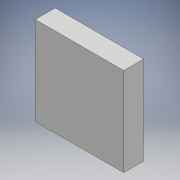
# Autodesk Inventor part: 球底座
Saved by Autodesk Inventor 2017 (Build 210142000, 142)
## iProperties
Created: 2021-05-18
Part Number: 球底座
Material: Generic
Document SubType Name: Modeling
Designer: user
Density: 1 g/cm^3
Appearance: Default
Author: user
Autodesk Inventor part; units mm, degrees
ref_plane "YZ Plane" through (0, 0, 0) normal (1, 0, 0) x (0, 1, 0)
ref_plane "XZ Plane" through (0, 0, 0) normal (0, 1, 0) x (-1, 0, 0)
sketch "Sketch1" plane through (0, 0, 0) normal (0, 1, 0) x (-1, 0, 0)
  line L0 (0, 0) -> (-400, 0)
  line L1 (-400, 0) -> (-400, -400)
  line L2 (-400, -400) -> (0, -400)
  line L3 (0, -400) -> (0, 0)
  dimension "d0" = 400
  dimension "d1" = 400
  constraints: 8 end point, 2 parallel, 1 horizontal, 1 perpendicular
  measures "d0" distance of L1.end L2.end
  measures "d1" distance of L2.end L0.start
extrude "Extrusion1" add sketch "Sketch1" along normal blind 20
ref_plane "Work Plane1" through (0, 0, -50) normal (0, 0, 1) x (1, 0, 0)
sketch "Sketch2" plane through (0, 0, -50) normal (0, 0, 1) x (1, 0, 0)
  line L0 (0, 20) -> (400, 20) projected
  arc A0 (4.9134, 69) -> (50, 25) centre (50, 70.1) ccw
  line L1 (50, 25) -> (50, 20)
  line L2 (0, 20) -> (50, 20)
  line L3 (50, 70.1) -> (50, 25)
  line L4 (0, 0) -> (0, 20) projected
  line L5 (0, 20) -> (0, 73.9134)
  line L6 (0, 73.9134) -> (4.9134, 69)
  dimension "d5" = 45.1
  dimension "d6" = 50
  dimension "d7" = 5
  dimension "d15" = 44
  dimension "d16" = 45
  constraints: 10 end point, 3 point on circle, 2 vertical, 1 centre point, 1 collinear, 1 perpendicular, 1 point on line
  measures "d5" radius of A0
  measures "d6" distance between parallel lines of L4 L1
  measures "d7" distance of L1.end L1.start
  measures "d15" vertical distance of L6.end L1.start
  measures "d16" angle of L5 L6
revolve "Revolution1" add sketch "Sketch2" angle 360 about axis through (50, 25, -50) along (0, -1, 0)
pattern_linear "Rectangular Pattern1" count 4 spacing 100 along (1, 0, 0) count 4 spacing -100 along (0, 0, 1) of "Revolution1"
sketch "Sketch4" plane through (0, 20, 0) normal (0, 1, 0) x (1, 0, 0)
  arc A0 (50, 100) -> (100, 150) centre (50, 150) ccw projected
  arc A1 (100, 50) -> (50, 100) centre (50, 50) ccw projected
  arc A2 (150, 100) -> (100, 50) centre (150, 50) ccw projected
  arc A3 (100, 150) -> (150, 100) centre (150, 150) ccw projected
  arc A4 (100, 250) -> (150, 200) centre (150, 250) ccw projected
  arc A5 (50, 200) -> (100, 250) centre (50, 250) ccw projected
  arc A6 (100, 150) -> (50, 200) centre (50, 150) ccw projected
  arc A7 (150, 200) -> (100, 150) centre (150, 150) ccw projected
  arc A8 (50, 200) -> (0, 150) centre (50, 150) ccw projected
  arc A9 (0, 250) -> (50, 200) centre (50, 250) ccw projected
  line L0 (0, 250) -> (0, 150) projected
  arc A10 (0, 150) -> (50, 100) centre (50, 150) ccw projected
  line L1 (0, 150) -> (0, 50) projected
  arc A11 (50, 100) -> (0, 50) centre (50, 50) ccw projected
  arc A12 (0, 50) -> (50, 0) centre (50, 50) ccw projected
  line L2 (0, 50) -> (0, 0) projected
  line L3 (0, 0) -> (50, 0) projected
  arc A13 (50, 300) -> (0, 250) centre (50, 250) ccw projected
  arc A14 (0, 350) -> (50, 300) centre (50, 350) ccw projected
  line L4 (0, 350) -> (0, 250) projected
  arc A15 (50, 400) -> (0, 350) centre (50, 350) ccw projected
  line L5 (50, 400) -> (0, 400) projected
  line L6 (0, 400) -> (0, 350) projected
  arc A16 (100, 350) -> (50, 400) centre (50, 350) ccw projected
  arc A17 (150, 400) -> (100, 350) centre (150, 350) ccw projected
  line L7 (150, 400) -> (50, 400) projected
  arc A18 (100, 350) -> (150, 300) centre (150, 350) ccw projected
  arc A19 (50, 300) -> (100, 350) centre (50, 350) ccw projected
  arc A20 (100, 250) -> (50, 300) centre (50, 250) ccw projected
  arc A21 (150, 300) -> (100, 250) centre (150, 250) ccw projected
  arc A22 (200, 350) -> (250, 300) centre (250, 350) ccw projected
  arc A23 (150, 300) -> (200, 350) centre (150, 350) ccw projected
  arc A24 (200, 250) -> (150, 300) centre (150, 250) ccw projected
  arc A25 (250, 300) -> (200, 250) centre (250, 250) ccw projected
  arc A26 (200, 250) -> (250, 200) centre (250, 250) ccw projected
  arc A27 (150, 200) -> (200, 250) centre (150, 250) ccw projected
  arc A28 (200, 150) -> (150, 200) centre (150, 150) ccw projected
  arc A29 (250, 200) -> (200, 150) centre (250, 150) ccw projected
  arc A30 (200, 150) -> (250, 100) centre (250, 150) ccw projected
  arc A31 (150, 100) -> (200, 150) centre (150, 150) ccw projected
  arc A32 (200, 50) -> (150, 100) centre (150, 50) ccw projected
  arc A33 (250, 100) -> (200, 50) centre (250, 50) ccw projected
  arc A34 (150, 0) -> (200, 50) centre (150, 50) ccw projected
  line L8 (150, 0) -> (250, 0) projected
  arc A35 (200, 50) -> (250, 0) centre (250, 50) ccw projected
  arc A36 (300, 150) -> (350, 100) centre (350, 150) ccw projected
  arc A37 (250, 100) -> (300, 150) centre (250, 150) ccw projected
  arc A38 (300, 50) -> (250, 100) centre (250, 50) ccw projected
  arc A39 (350, 100) -> (300, 50) centre (350, 50) ccw projected
  arc A40 (250, 0) -> (300, 50) centre (250, 50) ccw projected
  line L9 (250, 0) -> (350, 0) projected
  arc A41 (300, 50) -> (350, 0) centre (350, 50) ccw projected
  arc A42 (350, 0) -> (400, 50) centre (350, 50) ccw projected
  line L10 (350, 0) -> (400, 0) projected
  line L11 (400, 0) -> (400, 50) projected
  arc A43 (350, 100) -> (400, 150) centre (350, 150) ccw projected
  arc A44 (400, 50) -> (350, 100) centre (350, 50) ccw projected
  line L12 (400, 50) -> (400, 150) projected
  arc A45 (350, 200) -> (400, 250) centre (350, 250) ccw projected
  arc A46 (400, 150) -> (350, 200) centre (350, 150) ccw projected
  line L13 (400, 150) -> (400, 250) projected
  arc A47 (350, 200) -> (300, 150) centre (350, 150) ccw projected
  arc A48 (300, 250) -> (350, 200) centre (350, 250) ccw projected
  arc A49 (250, 200) -> (300, 250) centre (250, 250) ccw projected
  arc A50 (300, 150) -> (250, 200) centre (250, 150) ccw projected
  arc A51 (350, 300) -> (300, 250) centre (350, 250) ccw projected
  arc A52 (300, 350) -> (350, 300) centre (350, 350) ccw projected
  arc A53 (250, 300) -> (300, 350) centre (250, 350) ccw projected
  arc A54 (300, 250) -> (250, 300) centre (250, 250) ccw projected
  arc A55 (300, 350) -> (250, 400) centre (250, 350) ccw projected
  arc A56 (350, 400) -> (300, 350) centre (350, 350) ccw projected
  line L14 (350, 400) -> (250, 400) projected
  arc A57 (200, 350) -> (150, 400) centre (150, 350) ccw projected
  arc A58 (250, 400) -> (200, 350) centre (250, 350) ccw projected
  line L15 (250, 400) -> (150, 400) projected
  arc A59 (400, 350) -> (350, 400) centre (350, 350) ccw projected
  line L16 (400, 350) -> (400, 400) projected
  line L17 (400, 400) -> (350, 400) projected
  arc A60 (350, 300) -> (400, 350) centre (350, 350) ccw projected
  arc A61 (400, 250) -> (350, 300) centre (350, 250) ccw projected
  line L18 (400, 250) -> (400, 350) projected
  arc A62 (100, 50) -> (150, 0) centre (150, 50) ccw projected
  arc A63 (50, 0) -> (100, 50) centre (50, 50) ccw projected
  line L19 (50, 0) -> (150, 0) projected
extrude "Extrusion2" add sketch "Sketch4" along normal blind 48 contours A0 A3 A2 A1 | A11 L1 A10 | A6 A5 A4 A7 | A62 L19 A63 | L0 A9 A8 | A12 L3 L2 | A31 A30 A33 A32 | A27 A26 A29 A28 | A34 A35 L8 | L4 A14 A13 | A20 A19 A18 A21 | A24 A23 A22 A25 | A40 A41 L9 | L6 L5 A15 | A49 A48 A47 A50 | A37 A36 A39 A38 | A53 A52 A51 A54 | A42 L11 L10 | A16 L7 A17 | A57 L15 A58 | A55 L14 A56 | A43 L12 A44 | A45 L13 A46 | A60 L18 A61 | L17 L16 A59
sketch "Sketch5" plane through (0, 0, 0) normal (0, -1, 0) x (1, 0, 0)
  line L0 (-40, 40) -> (440, 40)
  line L1 (440, 40) -> (440, -440)
  line L2 (440, -440) -> (-40, -440)
  line L3 (-40, -440) -> (-40, 40)
  line L4 (400, 0) -> (400, -400) projected
  line L5 (400, -400) -> (0, -400) projected
  line L6 (0, 0) -> (400, 0) projected
  line L7 (0, -400) -> (0, 0) projected
  dimension "d20" = 40
  dimension "d21" = 40
  dimension "d22" = 40
  dimension "d23" = 40
  constraints: 8 end point, 2 parallel, 1 horizontal, 1 perpendicular
  measures "d20" distance between parallel lines of L1 L4
  measures "d21" distance between parallel lines of L2 L5
  measures "d22" distance between parallel lines of L0 L6
  measures "d23" distance between parallel lines of L3 L7
extrude "Extrusion3" add sketch "Sketch5" against normal up to surface (68 mm away)
sketch "Sketch6" plane through (0, 0, 0) normal (0, -1, 0) x (1, 0, 0)
  line L0 (-40, 40) -> (440, 40) projected
  line L1 (-40, -440) -> (-40, 40) projected
  line L2 (440, -440) -> (-40, -440) projected
  line L3 (440, 40) -> (440, -440) projected
  point P0 (0, 0)
extrude "Extrusion4" add sketch "Sketch6" along normal blind 40
body "Solid1"
